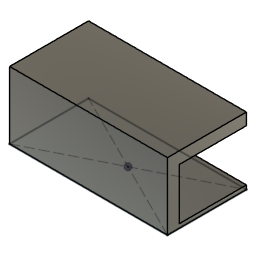
Hand Saw Mount (Autodesk Fusion 360 design; units mm, degrees)
Autodesk Fusion 360 part; units mm, degrees
sketch "Sketch1" plane through (0, 0, 0) normal (0, 0, 1) x (1, 0, 0)
  line L0 (20, -10) -> (-20, -10)
  line L1 (-20, -10) -> (-20, 10)
  line L2 (-20, 10) -> (20, 10)
  line L3 (20, 10) -> (20, -10)
  line L4 (20, -10) -> (-20, 10) construction
  line L5 (-20, -10) -> (20, 10) construction
  dimension "d1" = 40
  dimension "d2" = 20
  constraint horizontal L0
  constraint perpendicular L0 L1
  constraint parallel L0 L2
  constraint parallel L1 L3
  constraint coincident L4 origin
  constraint coincident L5 origin
  measures "d1" distance of L1 L3
  measures "d2" distance of L0 L2
extrude "Extrude1" add sketch "Sketch1" along normal blind 30
extrude "Extrude2" cut 1 faces at (6.6667, -3.3333, 30) along direction (0, 0, -1) blind 30
extrude "Extrude3" add sketch "Sketch1" along normal blind 17
sketch "Sketch2" plane through (0, 10, 0) normal (0, 1, 0) x (-1, 0, 0)
  line L0 (-20, 0) -> (20, 0)
  line L1 (20, 0) -> (20, 17)
  line L2 (20, 17) -> (-20, 17)
  line L3 (-20, 17) -> (-20, 0)
  line L4 (-20, 14) -> (20, 14)
  line L5 (20, 14) -> (20, 1)
  line L6 (20, 1) -> (-20, 1)
  line L7 (-20, 1) -> (-20, 14)
  dimension "d9" = 13
  constraint horizontal L4
  constraint vertical L5
  constraint horizontal L6
  constraint vertical L7
  constraint coincident L1 L5.end
  constraint coincident L3 L4.start
  measures "d9" distance of L4 L6
extrude "Extrude4" cut sketch "Sketch2" against normal blind 17 contours L1 L3 L4 L5 L6 L7
